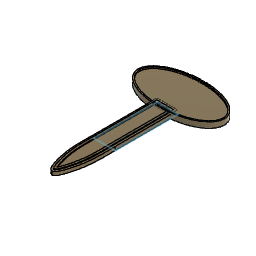
Rosen-Tafel v2 (Autodesk Fusion 360 design; units mm, degrees)
Autodesk Fusion 360 part; units mm, degrees
sketch "Skizze1" plane through (0, 0, 0) normal (0, 0, 1) x (1, 0, 0) in component "Tafe"
  ellipse E0 centre (0, 0) end of major axis (60, 0) minor radius 30
  line L0 (-60, 0) -> (60, 0)
  line L1 (0, -30) -> (0, 30)
  dimension "d1" = 60
  constraint coincident E0.centre origin
  constraint horizontal L0
  constraint coincident E0 L0.start
  constraint coincident E0 L0.end
  constraint coincident E0 L1.start
  constraint coincident E0 L1.end
  measures "d1" distance of E0
extrude "Extrusion1" add sketch "Skizze1" along normal blind 3 makes body 1 in component "Tafe"
sketch "Skizze2" plane through (0, 0, 3) normal (0, 0, 1) x (-1, 0, 0) in component "Tafe"
  ellipse E0 centre (0, 0) end of major axis (-60, 0) minor radius 30
  spline S0 degree 3 poles (61.9509, 0) (61.9509, 4.2635) (60.3055, 8.4828) (57.3091, 12.2636) (52.6449, 18.1488) (44.7166, 23.0684) (34.8255, 26.4973) (25.2136, 29.8294) (13.7584, 31.7256) (2.1658, 31.9316) (-9.8896, 32.1459) (-22.0459, 30.5274) (-32.3487, 27.3124) (-41.3637, 24.4992) (-48.9522, 20.4892) (-54.1681, 15.6411) (-58.1005, 11.9859) (-60.7028, 7.8251) (-61.5993, 3.4465) (-62.4053, -0.4903) (-61.7899, -4.5541) (-59.8722, -8.3093) (-56.3973, -15.1137) (-48.7697, -20.9418) (-38.5998, -25.0786) (-29.6788, -28.7075) (-18.796, -31.0188) (-7.5068, -31.7189) (4.0223, -32.434) (15.9353, -31.462) (26.4461, -28.9362) (36.7725, -26.4548) (45.7187, -22.4959) (52.0049, -17.4981) (56.4978, -13.926) (59.6597, -9.8063) (61.0885, -5.3839) (61.6588, -3.6187) (61.9509, -1.8099) (61.9509, 0) knots -3.141593 -3.141593 -3.141593 -3.141593 -2.764311 -2.764311 -2.764311 -2.177028 -2.177028 -2.177028 -1.606323 -1.606323 -1.606323 -1.012833 -1.012833 -1.012833 -0.49353 -0.49353 -0.49353 -0.102016 -0.102016 -0.102016 0.249996 0.249996 0.249996 0.887852 0.887852 0.887852 1.447382 1.447382 1.447382 2.018805 2.018805 2.018805 2.580199 2.580199 2.580199 2.981436 2.981436 2.981436 3.141593 3.141593 3.141593 3.141593
  dimension "d4" = 1.9509
extrude "Extrusion2" add sketch "Skizze2" along normal blind 2 and the other way blind 2 bodies 1 in component "Tafe"
sketch "Skizze3" plane through (0, 0, 0) normal (0, 0, 1) x (1, 0, 0) in component "Tafe"
extrude "Extrusion3" add 1 faces at (23.0091, -28.1834, 1) along direction (0, 0, -1) blind 1 on bodies 1 bodies 1 in component "Tafe"
sketch "Skizze1 (2)" plane through (0, 0, 0) normal (0, 0, 1) x (1, 0, 0) in component "Ständer"
extrude "Extrusion4" add 2 faces at (23.0091, -28.1834, 0) (8.4972, -9.7981, 0) along direction (0, 0, -1) blind 3 on bodies 1 bodies 1 in component "Tafe"
sketch "Skizze2 (2)" plane through (0, 0, -3) normal (0, 0, -1) x (1, 0, 0) in component "Ständer"
  spline S0 degree 3 poles (-61.9509, 0) (-61.9509, -1.8099) (-61.6588, -3.6187) (-61.0885, -5.3839) (-59.6597, -9.8063) (-56.4978, -13.926) (-52.0049, -17.4981) (-45.7187, -22.4959) (-36.7725, -26.4548) (-26.4461, -28.9362) (-15.9353, -31.462) (-4.0223, -32.434) (7.5068, -31.7189) (18.796, -31.0188) (29.6788, -28.7075) (38.5998, -25.0786) (48.7697, -20.9418) (56.3973, -15.1137) (59.8722, -8.3093) (61.7899, -4.5541) (62.4053, -0.4903) (61.5993, 3.4465) (60.7028, 7.8251) (58.1005, 11.9859) (54.1681, 15.6411) (48.9522, 20.4892) (41.3637, 24.4992) (32.3487, 27.3124) (22.0459, 30.5274) (9.8896, 32.1459) (-2.1658, 31.9316) (-13.7584, 31.7256) (-25.2136, 29.8294) (-34.8255, 26.4973) (-44.7166, 23.0684) (-52.6449, 18.1488) (-57.3091, 12.2636) (-60.3055, 8.4828) (-61.9509, 4.2635) (-61.9509, 0) knots -3.141593 -3.141593 -3.141593 -3.141593 -2.981436 -2.981436 -2.981436 -2.580199 -2.580199 -2.580199 -2.018805 -2.018805 -2.018805 -1.447382 -1.447382 -1.447382 -0.887852 -0.887852 -0.887852 -0.249996 -0.249996 -0.249996 0.102016 0.102016 0.102016 0.49353 0.49353 0.49353 1.012833 1.012833 1.012833 1.606323 1.606323 1.606323 2.177028 2.177028 2.177028 2.764311 2.764311 2.764311 3.141593 3.141593 3.141593 3.141593
  line L0 (15, 20) -> (-15, 20)
  line L1 (-15, 20) -> (-15, 110)
  line L2 (-15, 110) -> (15, 110)
  line L3 (15, 110) -> (15, 20)
  constraint horizontal L0
  constraint vertical L1
  constraint horizontal L2
  constraint vertical L3
extrude "Extrusion1'" add sketch "Skizze2 (2)" against normal blind 5 separate body contours S0 L0 L1 L3 picked at (1.6815, 23.9477) makes body 2 in component "Ständer"
extrude "Extrusion2'" add sketch "Skizze2 (2)" against normal blind 5 contours S0 L1 L2 L3 bodies 2 in component "Ständer"
sketch "Skizze3 (2)" plane through (0, 0, 2) normal (0, 0, 1) x (-1, 0, 0) in component "Ständer"
  line L0 (15, 20) -> (15, 110)
  line L1 (15, 110) -> (-15, 110)
  line L2 (-15, 110) -> (-15, 20)
  line L3 (-15, 20) -> (15, 20)
  spline S0 degree 5 poles (15, 110) (15.0176, 110.8619) (15.0503, 112.5708) (15.0915, 115.0899) (15.1309, 118.3598) (15.1537, 122.2987) (15.1484, 126.0898) (15.1122, 129.7366) (15.0406, 133.2467) (14.9275, 136.6331) (14.7639, 139.9163) (14.5397, 143.1226) (14.2439, 146.2818) (13.867, 149.4242) (13.4012, 152.5784) (12.8426, 155.769) (12.1915, 159.0132) (11.4507, 162.3163) (10.6251, 165.6668) (9.72, 169.0317) (8.7408, 172.3517) (7.6913, 175.5347) (6.574, 178.4677) (5.3908, 181.0335) (4.1426, 183.1253) (2.8302, 184.6621) (1.7296, 185.4171) (0.8758, 185.7125) (0.294, 185.7893) (0, 185.7977) knots 0 0 0 0 0 0 0.04 0.08 0.12 0.16 0.2 0.24 0.28 0.32 0.36 0.4 0.44 0.48 0.52 0.56 0.6 0.64 0.68 0.72 0.76 0.8 0.84 0.88 0.92 0.96 1 1 1 1 1 1
  line L4 (0, -2.5) -> (0, -20)
  spline S1 degree 5 poles (-15, 110) (-15.0176, 110.8619) (-15.0503, 112.5708) (-15.0915, 115.0899) (-15.1309, 118.3598) (-15.1537, 122.2987) (-15.1484, 126.0898) (-15.1122, 129.7366) (-15.0406, 133.2467) (-14.9275, 136.6331) (-14.7639, 139.9163) (-14.5397, 143.1226) (-14.2439, 146.2818) (-13.867, 149.4242) (-13.4012, 152.5784) (-12.8426, 155.769) (-12.1915, 159.0132) (-11.4507, 162.3163) (-10.6251, 165.6668) (-9.72, 169.0317) (-8.7408, 172.3517) (-7.6913, 175.5347) (-6.574, 178.4677) (-5.3908, 181.0335) (-4.1426, 183.1253) (-2.8302, 184.6621) (-1.7296, 185.4171) (-0.8758, 185.7125) (-0.294, 185.7893) (0, 185.7977) knots 0 0 0 0 0 0 0.04 0.08 0.12 0.16 0.2 0.24 0.28 0.32 0.36 0.4 0.44 0.48 0.52 0.56 0.6 0.64 0.68 0.72 0.76 0.8 0.84 0.88 0.92 0.96 1 1 1 1 1 1
  line L5 (14.8117, 100.8471) -> (15.1883, 119.1529)
  line L6 (6.7737, 185.6047) -> (-6.7737, 185.9906)
  line L7 (-14.8117, 100.8471) -> (-15.1883, 119.1529)
  line L8 (-6.7737, 185.6047) -> (6.7737, 185.9906)
  point P0 (15, 134.2579)
  point P1 (13.5579, 151.4378)
  point P2 (9.54, 169.5876)
  point P3 (3.9981, 183.1652)
  point P4 (-15, 134.2579)
  point P5 (-13.5579, 151.4378)
  point P6 (-9.54, 169.5876)
  point P7 (-3.9981, 183.1652)
  constraint coincident L0.end L1.start
  constraint midpoint L0.end L5
  constraint midpoint S0.end L6
  constraint symmetric L0.end L4 L1.end
  constraint symmetric P0 L4 P4
  constraint symmetric P1 L4 P5
  constraint symmetric P2 L4 P6
  constraint symmetric P3 L4 P7
  constraint symmetric S0.end L4 S1.end
  constraint symmetric L4 L5.start L7.start
  constraint symmetric L4 L5.end L7.end
  constraint symmetric L4 L6.start L8.start
  constraint symmetric L4 L6.end L8.end
extrude "Extrusion3'" add sketch "Skizze3 (2)" against normal blind 5 contours L1 S0 S1 bodies 2 in component "Ständer"
sketch "Skizze4" plane through (0, 0, 2) normal (0, 0, 1) x (-1, 0, 0) in component "Ständer"
  line L0 (15, 20) -> (15, 110)
  spline S0 degree 5 poles (15, 110) (15.0176, 110.8619) (15.0503, 112.5708) (15.0915, 115.0899) (15.1309, 118.3598) (15.1537, 122.2987) (15.1484, 126.0898) (15.1122, 129.7366) (15.0406, 133.2467) (14.9275, 136.6331) (14.7639, 139.9163) (14.5397, 143.1226) (14.2439, 146.2818) (13.867, 149.4242) (13.4012, 152.5784) (12.8426, 155.769) (12.1915, 159.0132) (11.4507, 162.3163) (10.6251, 165.6668) (9.72, 169.0317) (8.7408, 172.3517) (7.6913, 175.5347) (6.574, 178.4677) (5.3908, 181.0335) (4.1426, 183.1253) (2.8302, 184.6621) (1.7296, 185.4171) (0.8758, 185.7125) (0.294, 185.7893) (0, 185.7977) knots 0 0 0 0 0 0 0.04 0.08 0.12 0.16 0.2 0.24 0.28 0.32 0.36 0.4 0.44 0.48 0.52 0.56 0.6 0.64 0.68 0.72 0.76 0.8 0.84 0.88 0.92 0.96 1 1 1 1 1 1
  spline S1 degree 5 poles (-15, 110) (-15.0176, 110.8619) (-15.0503, 112.5708) (-15.0915, 115.0899) (-15.1309, 118.3598) (-15.1537, 122.2987) (-15.1484, 126.0898) (-15.1122, 129.7366) (-15.0406, 133.2467) (-14.9275, 136.6331) (-14.7639, 139.9163) (-14.5397, 143.1226) (-14.2439, 146.2818) (-13.867, 149.4242) (-13.4012, 152.5784) (-12.8426, 155.769) (-12.1915, 159.0132) (-11.4507, 162.3163) (-10.6251, 165.6668) (-9.72, 169.0317) (-8.7408, 172.3517) (-7.6913, 175.5347) (-6.574, 178.4677) (-5.3908, 181.0335) (-4.1426, 183.1253) (-2.8302, 184.6621) (-1.7296, 185.4171) (-0.8758, 185.7125) (-0.294, 185.7893) (0, 185.7977) knots 0 0 0 0 0 0 0.04 0.08 0.12 0.16 0.2 0.24 0.28 0.32 0.36 0.4 0.44 0.48 0.52 0.56 0.6 0.64 0.68 0.72 0.76 0.8 0.84 0.88 0.92 0.96 1 1 1 1 1 1
  line L1 (-15, 110) -> (-15, 20)
  line L2 (-15, 20) -> (15, 20)
  spline S2 degree 3 poles (-11.9777, 110.0309) (-11.9779, 110.0412) (-11.9781, 110.0515) (-11.9783, 110.0618) (-12.1467, 118.2962) (-12.1876, 125.6884) (-12.0304, 132.2915) (-11.8915, 138.1249) (-11.5879, 143.3276) (-10.915, 148.5264) (-10.4464, 152.1476) (-9.7926, 155.8041) (-8.949, 159.6156) (-8.1726, 163.1233) (-7.2391, 166.7794) (-6.1929, 170.2595) (-5.0109, 174.1918) (-3.6533, 177.8638) (-2.3593, 180.1318) (-1.7058, 181.2772) (-1.0734, 182.0403) (-0.6357, 182.4064) (-0.297, 182.6897) (-0.1153, 182.7456) (0, 182.7673) knots -0.000287 -0.000287 -0.000287 -0.000287 0 0 0 0.23016 0.23016 0.23016 0.433487 0.433487 0.433487 0.575116 0.575116 0.575116 0.705456 0.705456 0.705456 0.852728 0.852728 0.852728 0.927106 0.927106 0.927106 0.984664 0.984664 0.984664 0.984664
  spline S3 degree 3 poles (11.9777, 110.0309) (11.9779, 110.0412) (11.9781, 110.0515) (11.9783, 110.0618) (12.1467, 118.2962) (12.1876, 125.6884) (12.0304, 132.2915) (11.8915, 138.1249) (11.5879, 143.3276) (10.915, 148.5264) (10.4464, 152.1476) (9.7926, 155.8041) (8.949, 159.6156) (8.1726, 163.1233) (7.2391, 166.7794) (6.1929, 170.2595) (5.0109, 174.1918) (3.6533, 177.8638) (2.3593, 180.1318) (1.7058, 181.2772) (1.0734, 182.0403) (0.6357, 182.4064) (0.297, 182.6897) (0.1153, 182.7456) (0, 182.7673) knots -0.000287 -0.000287 -0.000287 -0.000287 0 0 0 0.23016 0.23016 0.23016 0.433487 0.433487 0.433487 0.575116 0.575116 0.575116 0.705456 0.705456 0.705456 0.852728 0.852728 0.852728 0.927106 0.927106 0.927106 0.984664 0.984664 0.984664 0.984664
  line L3 (11.9777, 23.0223) -> (11.9777, 110.0309)
  line L4 (-11.9777, 23.0223) -> (11.9777, 23.0223)
  line L5 (-11.9777, 110.0309) -> (-11.9777, 23.0223)
  spline S4 degree 3 poles (-9, 110.0613) (-9.0004, 110.0818) (-9.0008, 110.1022) (-9.0013, 110.1226) (-9.1708, 118.4153) (-9.2103, 125.8461) (-9.0484, 132.4316) (-8.9146, 137.8751) (-8.6346, 142.7164) (-8.0427, 147.5055) (-7.6174, 150.9474) (-7.0241, 154.4041) (-6.2475, 158.0272) (-5.5493, 161.2843) (-4.705, 164.6878) (-3.7598, 167.9778) (-2.8347, 171.1978) (-1.801, 174.2968) (-0.8034, 176.5706) (-0.5276, 177.1992) (-0.2561, 177.763) (0, 178.2439) knots -0.000569 -0.000569 -0.000569 -0.000569 0 0 0 0.232641 0.232641 0.232641 0.424939 0.424939 0.424939 0.56314 0.56314 0.56314 0.687378 0.687378 0.687378 0.80897 0.80897 0.80897 0.842587 0.842587 0.842587 0.842587
  spline S5 degree 3 poles (9, 110.0613) (9.0004, 110.0818) (9.0008, 110.1022) (9.0013, 110.1226) (9.1708, 118.4153) (9.2103, 125.8461) (9.0484, 132.4316) (8.9146, 137.8751) (8.6346, 142.7164) (8.0427, 147.5055) (7.6174, 150.9474) (7.0241, 154.4041) (6.2475, 158.0272) (5.5493, 161.2843) (4.705, 164.6878) (3.7598, 167.9778) (2.8347, 171.1978) (1.801, 174.2968) (0.8034, 176.5706) (0.5276, 177.1992) (0.2561, 177.763) (0, 178.2439) knots -0.000569 -0.000569 -0.000569 -0.000569 0 0 0 0.232641 0.232641 0.232641 0.424939 0.424939 0.424939 0.56314 0.56314 0.56314 0.687378 0.687378 0.687378 0.80897 0.80897 0.80897 0.842587 0.842587 0.842587 0.842587
  line L6 (9, 26) -> (9, 110.0613)
  line L7 (-9, 26) -> (9, 26)
  line L8 (-9, 110.0613) -> (-9, 26)
  dimension "d19" = -3.0223
  dimension "d20" = -6
extrude "Extrusion4'" add sketch "Skizze4" along normal blind 1 contours S2 S3 L3 L4 L5 bodies 2 in component "Ständer"
component "Tafe" placed x (1, 0, 0) y (0, 1, 0) z (0, 0, 1) at (0, 0, 0)
component "Ständer" placed x (1, 0, 0) y (0, 1, 0) z (0, 0, 1) at (0, 0, 0)
named bodies: "Grundplatte"
